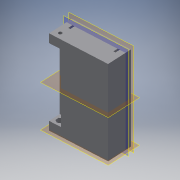
# Autodesk Inventor part: Caixa Painel
Saved by Autodesk Inventor 2019 (Build 230136000, 136)
## iProperties
Created: 2020-05-29
Part Number: Caixa Painel
Material: Generic
Document SubType Name: Modeling
Designer: luiza
Density: 1 g/cm^3
Appearance: Default
Categories: <MemberInstance><Categories><Category DisplayName="" Mnemonic="CABLEANDHARNESS" InternalName="e4a7e005-5e42-4d16-b293-125e7f0d0512"><Category DisplayName="" Mnemonic="CONNECTORS" InternalName="6f634eba-a678-4820-a31d-2c2d5ee6728e"><CategoryParameter DisplayName="" Mnemonic="REFDES" InternalName="c3740e8c-60ab-4d5d-8584-52b73222f2f0"/><Category DisplayName="" Mnemonic="DISCRETEWIRE" InternalName="9a3407de-09b2-4cdb-8c40-9708d5144a28"/></Category></Category></Categories><FamilyTemplate><FamilyTemplateParameters></FamilyTemplateParameters></FamilyTemplate><CategoryParameterMap><ParamToTemplateMap><ParamToTemplate CategoryParameter="//CategoryParameter[@InternalName='c3740e8c-60ab-4d5d-8584-52b73222f2f0']" ConstantValue=""/></ParamToTemplateMap></CategoryParameterMap></MemberInstance>
Author: luiza
Autodesk Inventor part; units mm, degrees
ref_plane "YZ Plane" through (0, 0, 0) normal (1, 0, 0) x (0, 1, 0)
ref_plane "XZ Plane" through (0, 0, 0) normal (0, 1, 0) x (-1, 0, 0)
ref_plane "XY Plane" through (0, 0, 0) normal (0, 0, 1) x (1, 0, 0)
ref_plane "Work Plane1" through (-1405.2046, 1188.2554, 32.7938) normal (0.0525168, 0, 0.99862) x (0, -1, 0)
sketch "Sketch1" plane through (-1405.2046, 1188.2554, 32.7938) normal (0.0525168, 0, 0.99862) x (0, -1, 0)
  line L0 (-58, 47) -> (58, 47)
  line L1 (72, 33) -> (72, -33)
  line L2 (58, -47) -> (-58, -47)
  line L3 (-72, -33) -> (-72, 33)
  line L4 (-65, 33) -> (-72, 33)
  line L5 (-58, 40) -> (-58, 47)
  arc A0 (-65, 33) -> (-58, 40) centre (-65, 40) ccw
  line L6 (0, 69.334) -> (0, -92.7299)
  line L7 (101.325, 0) -> (-113.3608, 0)
  line L8 (65, 33) -> (72, 33)
  line L9 (58, 40) -> (58, 47)
  arc A1 (58, 40) -> (65, 33) centre (65, 40) ccw
  line L10 (-65, -33) -> (-72, -33)
  line L11 (-58, -40) -> (-58, -47)
  arc A2 (-58, -40) -> (-65, -33) centre (-65, -40) ccw
  line L12 (58, -40) -> (58, -47)
  arc A3 (65, -33) -> (58, -40) centre (65, -40) ccw
  line L13 (65, -33) -> (72, -33)
  line L14 (75, -50) -> (75, 50)
  line L15 (75, 50) -> (-75, 50)
  line L16 (-75, 50) -> (-75, -50)
  line L17 (-75, -50) -> (75, -50)
  constraints: 36 end point, 15 symmetric about line, 8 point on circle, 4 centre point, 4 horizontal, 4 vertical, 1 coincident, 7 other
extrude "Extrusion1" add sketch "Sketch1" along normal blind 40 contours L5 A0 L4 L3 L7 L16 L15 L6 L0 | L6 L15 L14 L7 L1 L8 A1 L9 L0 | L6 L17 L16 L7 L3 L10 A2 L11 L2 | L2 L12 A3 L13 L1 L7 L14 L17 L6
sketch "Sketch2" plane through (-1403.1039, 1188.2554, 72.7386) normal (0.0525168, 0, 0.99862) x (0, -1, 0)
  line L0 (72, -33) -> (65, -33) projected
  arc A0 (65, -33) -> (58, -40) centre (65, -40) ccw projected
  line L1 (58, -40) -> (58, -47) projected
  line L2 (58, -47) -> (-58, -47) projected
  line L3 (-58, -47) -> (-58, -40) projected
  arc A1 (-58, -40) -> (-65, -33) centre (-65, -40) ccw projected
  line L4 (-65, -33) -> (-72, -33) projected
  line L5 (-72, -33) -> (-72, 33) projected
  line L6 (-72, 33) -> (-65, 33) projected
  arc A2 (-65, 33) -> (-58, 40) centre (-65, 40) ccw projected
  line L7 (-58, 40) -> (-58, 47) projected
  line L8 (-58, 47) -> (58, 47) projected
  line L9 (58, 47) -> (58, 40) projected
  arc A3 (58, 40) -> (65, 33) centre (65, 40) ccw projected
  line L10 (65, 33) -> (72, 33) projected
  line L11 (72, 33) -> (72, -33) projected
  line L12 (-75, 50) -> (75, 50)
  line L13 (75, 50) -> (75, -50)
  line L14 (75, -50) -> (-75, -50)
  line L15 (-75, -50) -> (-75, 50)
  point P0 (75, -40)
  constraints: 8 end point, 2 horizontal, 2 vertical, 4 other
extrude "Extrusion2" add sketch "Sketch2" along normal blind 3 contours L0 A0 L1 L2 L3 A1 L4 L5 L6 A2 L7 L8 L9 A3 L10 L11 | L12 L13 L14 L15
ref_plane "Work Plane2" through (-1404.6794, 1188.2554, 42.78) normal (-0.0525168, 0, -0.99862) x (0, -1, 0)
sketch "Sketch3" plane through (-1404.6794, 1188.2554, 42.78) normal (-0.0525168, 0, -0.99862) x (0, -1, 0)
  line L0 (72, -33) -> (72, 33) projected
  line L1 (-58, -47) -> (58, -47) projected
  line L2 (72, 0) -> (-85.4188, 0)
  line L3 (0, -47) -> (0, 56.7085)
  line L4 (-67.1246, 36.5) -> (-63.0716, 36.4992)
  line L5 (-69.1504, 40.0104) -> (-67.1246, 36.5) construction
  line L6 (-67.1232, 43.52) -> (-69.1504, 40.0104) construction
  line L7 (-63.0702, 43.5192) -> (-67.1232, 43.52)
  line L8 (-63.0716, 36.4992) -> (-61.0444, 40.0088)
  line L9 (-61.0444, 40.0088) -> (-63.0702, 43.5192)
  line L10 (-61.0444, 40.0088) -> (-77.9922, 40.0088)
  line L11 (-64.8068, 40.0088) -> (-83.3652, 40.0088) construction
  line L12 (-67.1232, 43.52) -> (-74.36, 43.52)
  line L13 (-67.1246, 36.5) -> (-75, 36.5)
  arc A0 (74.36, -43.52) -> (75, -40) centre (65, -40) ccw
  arc A1 (-75, -40) -> (-74.36, -43.52) centre (-65, -40) ccw
  arc A2 (-74.36, 43.52) -> (-75, 40) centre (-65, 40) ccw
  arc A3 (75, 40) -> (74.36, 43.52) centre (65, 40) ccw
  line L14 (63.0716, 36.4992) -> (61.0444, 40.0088)
  line L15 (61.0444, 40.0088) -> (63.0702, 43.5192)
  line L16 (69.1504, 40.0104) -> (67.1246, 36.5) construction
  line L17 (67.1232, 43.52) -> (69.1504, 40.0104) construction
  line L18 (67.1246, 36.5) -> (63.0716, 36.4992)
  line L19 (63.0702, 43.5192) -> (67.1232, 43.52)
  line L20 (61.0444, 40.0088) -> (77.9922, 40.0088)
  line L21 (67.1232, 43.52) -> (74.36, 43.52)
  line L22 (67.1246, 36.5) -> (75, 36.5)
  line L23 (-63.0716, -36.4992) -> (-61.0444, -40.0088)
  line L24 (-61.0444, -40.0088) -> (-63.0702, -43.5192)
  line L25 (-69.1504, -40.0104) -> (-67.1246, -36.5) construction
  line L26 (-67.1232, -43.52) -> (-69.1504, -40.0104) construction
  line L27 (-67.1246, -36.5) -> (-63.0716, -36.4992)
  line L28 (-63.0702, -43.5192) -> (-67.1232, -43.52)
  line L29 (-61.0444, -40.0088) -> (-77.9922, -40.0088)
  line L30 (-67.1232, -43.52) -> (-74.36, -43.52)
  line L31 (-67.1246, -36.5) -> (-75, -36.5)
  line L32 (63.0716, -36.4992) -> (61.0444, -40.0088)
  line L33 (61.0444, -40.0088) -> (63.0702, -43.5192)
  line L34 (69.1504, -40.0104) -> (67.1246, -36.5) construction
  line L35 (67.1246, -36.5) -> (63.0716, -36.4992)
  line L36 (63.0702, -43.5192) -> (67.1232, -43.52)
  line L37 (67.1232, -43.52) -> (69.1504, -40.0104) construction
  line L38 (67.1246, -36.5) -> (75, -36.5)
  line L39 (67.1232, -43.52) -> (74.36, -43.52)
  line L40 (61.0444, -40.0088) -> (77.9922, -40.0088)
  line L41 (-75, -40) -> (-75, -36.5)
  line L42 (-75, 36.5) -> (-75, 40)
  line L43 (75, 40) -> (75, 36.5)
  line L44 (75, -36.5) -> (75, -40)
  point P0 (1188.2554, -1404.9877)
  point P1 (64.8068, 40.0088)
  point P2 (-64.8068, -40.0088)
  point P3 (-65, -40)
  point P4 (65, -40)
  point P5 (64.8068, -40.0088)
  point P6 (65, -40)
  dimension "d27" = 7.02
  dimension "d28" = 7.02
  dimension "d29" = 7.02
  constraints: 86 end point, 34 symmetric about line, 8 point on circle, 7 centre point, 6 horizontal, 4 equal length, 2 midpoint, 2 parallel, 1 collinear, 1 vertical
  measures "d27" distance between parallel lines of L4 L7
  measures "d28" distance between parallel lines of L9 L5
  measures "d29" distance between parallel lines of L6 L8
extrude "Extrusion5" cut sketch "Sketch3" against normal blind 8
sketch "Sketch4" plane through (-1405.2046, 1188.2554, 32.7938) normal (-0.0525168, 0, -0.99862) x (0, -1, 0)
  line L0 (65, 33) -> (72, 33) projected
  line L1 (72, 33) -> (72, -33) projected
  line L2 (72, -33) -> (65, -33) projected
  arc A0 (65, -33) -> (58, -40) centre (65, -40) ccw projected
  line L3 (58, -40) -> (58, -47) projected
  line L4 (58, -47) -> (-58, -47) projected
  line L5 (-58, -47) -> (-58, -40) projected
  arc A1 (-58, -40) -> (-65, -33) centre (-65, -40) ccw projected
  line L6 (-65, -33) -> (-72, -33) projected
  line L7 (-72, -33) -> (-72, 33) projected
  line L8 (-72, 33) -> (-65, 33) projected
  arc A2 (-65, 33) -> (-58, 40) centre (-65, 40) ccw projected
  line L9 (-58, 40) -> (-58, 47) projected
  line L10 (-58, 47) -> (58, 47) projected
  line L11 (58, 47) -> (58, 40) projected
  arc A3 (58, 40) -> (65, 33) centre (65, 40) ccw projected
  circle A4 centre (-65, 40) radius 2
  circle A5 centre (65, 40) radius 2
  circle A6 centre (65, -40) radius 2
  circle A7 centre (-65, -40) radius 2
  point P0 (1188.2554, -1404.9877)
  dimension "d19" = 4
  dimension "d20" = 4
  dimension "d21" = 4
  dimension "d22" = 4
  constraints: 4 centre point
  measures "d19" diameter of A7
  measures "d20" diameter of A4
  measures "d21" diameter of A5
  measures "d22" diameter of A6
extrude "Extrusion6" cut sketch "Sketch4" against normal blind 24 contours A4 | A5 | A6 | A7
sketch "Sketch15" plane through (-1455.1356, 1113.2554, 35.4196) normal (0, -1, 0) x (0.99862, 0, -0.0525168)
  circle A0 centre (10, 33) radius 3
  line L0 (0, 40) -> (100, 40) projected
  line L1 (0, 0) -> (0, 40) projected
  point P0 (1454.9877, 41.0484)
  dimension "d74" = 7
  dimension "d75" = 6
  dimension "d76" = 10
  constraints: 1 centre point
  measures "d74" distance from line of L0 A0.centre
  measures "d75" diameter of A0
  measures "d76" distance from line of L1 A0.centre
extrude "Extrusion14" cut sketch "Sketch15" against normal through all
ref_plane "Work Plane7" through (-1438.1591, 1114.7554, 34.5268) normal (0, 1, 0) x (0.99862, 0, -0.0525168)
sketch "Sketch16" plane through (-1438.1591, 1114.7554, 34.5268) normal (0, 1, 0) x (0.99862, 0, -0.0525168)
  line L0 (-17, 0) -> (-17, -43) projected
  line L1 (-17, -43) -> (3, -43)
  line L2 (3, -43) -> (3, -23)
  line L3 (3, -23) -> (-17, -23)
  line L4 (-17, -23) -> (-17, -43)
  circle A0 centre (-7, -33) radius 3 projected
  dimension "d79" = 10
  dimension "d80" = 10
  constraints: 8 end point, 2 parallel, 1 horizontal, 1 perpendicular
  measures "d79" distance from line of L2 A0.centre
  measures "d80" distance from line of L3 A0.centre
extrude "Extrusion15" cut sketch "Sketch16" along normal up to surface (145.5 mm away)
sketch "Sketch17" plane through (-1438.1591, 1260.2554, 34.5268) normal (0, -1, 0) x (0.99862, 0, -0.0525168)
  line L0 (-17, 43) -> (3, 43) projected
  line L1 (-17, 23) -> (-17, 43) projected
  line L2 (-7, 23) -> (-14, 23) projected
  line L3 (3, 40) -> (3, 43) projected
  line L4 (3, 43) -> (3, 23)
  line L5 (-17, 23) -> (3, 23)
  line L6 (8, 18) -> (-17, 18)
  line L7 (8, 43) -> (8, 18)
  line L8 (83, 43) -> (-17, 43) projected
  line L9 (8, 43) -> (3, 43)
  line L10 (-17, 23) -> (-17, 18)
  line L11 (-17, 0) -> (-17, 43) projected
  dimension "d83" = 5
  constraints: 12 end point, 2 point on line, 1 collinear, 1 horizontal, 1 vertical
  measures "d83" distance between parallel lines of L4 L7
extrude "Extrusion16" add sketch "Sketch17" along normal up to surface (144 mm away) contours L8 L7 L6 L10 L5 L2 L4 L3
sketch "Sketch18" plane through (-1433.9553, 1260.2554, 57.3375) normal (0, -1, 0) x (0.99862, 0, -0.0525168)
  circle A0 centre (-10, 10) radius 3 projected
  circle A1 centre (-10, 10) radius 6.3509 construction
  line L0 (-10, 16.3509) -> (-4.5, 13.1754)
  line L1 (-4.5, 13.1754) -> (-4.5, 6.8246)
  line L2 (-4.5, 6.8246) -> (-10, 3.6491)
  line L3 (-10, 3.6491) -> (-15.5, 6.8246)
  line L4 (-15.5, 6.8246) -> (-15.5, 13.1754)
  line L5 (-15.5, 13.1754) -> (-10, 16.3509)
  line L6 (-15.5, 10) -> (-4.5, 10)
  line L7 (0, 0) -> (0, 20) projected
  line L8 (-20, 20) -> (0, 20) projected
  line L9 (-20, 0) -> (-20, 20) projected
  line L10 (-20, 0) -> (0, 0) projected
  circle A2 centre (-10, 10) radius 3 projected
  dimension "d89" = 11
  constraints: 14 end point, 6 point on circle, 3 equal length, 2 midpoint, 2 vertical, 1 centre point, 1 coincident, 1 parallel
  measures "d89" distance of L6.start L6.end
extrude "Extrusion17" add sketch "Sketch18" along normal blind 12
ref_plane "Work Plane8" through (-1455.1356, 1188.2554, 35.4196) normal (0, 1, 0) x (0.99862, 0, -0.0525168)
mirror "Mirror4" about plane through (-1455.1356, 1188.2554, 35.4196) normal (0, 1, 0) of "Extrusion17"
sketch "Sketch19" plane through (-1438.1591, 1114.7554, 34.5268) normal (0, 1, 0) x (0.99862, 0, -0.0525168)
  circle A0 centre (-7, -33) radius 3 projected
  line L0 (3, -43) -> (-17, -43) projected
  line L1 (3, -43) -> (3, -23) projected
  line L2 (3, -23) -> (-17, -23) projected
  line L3 (-17, -43) -> (-17, -23) projected
  point P0 (1437.9877, -41.0484)
extrude "Extrusion18" add sketch "Sketch19" along normal up to surface (1.5 mm away)
sketch "Sketch20" plane through (-1433.9553, 1128.2554, 57.3375) normal (0.0525168, 0, 0.99862) x (0.99862, 0, -0.0525168)
  arc A0 (-3.75, 66.129) -> (-13.25, 66.129) centre (-8.5, 66.129) ccw
  arc A1 (-13.25, 53.871) -> (-3.75, 53.871) centre (-8.5, 53.871) ccw
  line L0 (-3.75, 66.129) -> (-3.75, 53.871)
  line L1 (-13.25, 66.129) -> (-13.25, 53.871)
  line L2 (-20, 0) -> (0, 0) projected
  line L3 (0, 0) -> (0, 120) projected
  line L4 (0, 120) -> (-20, 120) projected
  line L5 (-20, 0) -> (-20, 120) projected
  line L6 (-17, 118) -> (-17, 2) projected
  line L7 (-17, 60) -> (0, 60)
  line L8 (-17, 118) -> (0, 118)
  line L9 (-8.5, 118) -> (-8.5, 0)
  line L10 (-3.75, 60) -> (-13.25, 60)
  line L11 (-8.5, 70.879) -> (-8.5, 49.121)
  arc A2 (-3.75, 93.387) -> (-13.25, 93.387) centre (-8.5, 93.387) ccw
  arc A3 (-13.25, 81.129) -> (-3.75, 81.129) centre (-8.5, 81.129) ccw
  line L12 (-3.75, 93.387) -> (-3.75, 81.129)
  line L13 (-13.25, 93.387) -> (-13.25, 81.129)
  line L14 (-3.75, 87.258) -> (-13.25, 87.258)
  line L15 (-8.5, 98.137) -> (-8.5, 76.379)
  arc A4 (-3.75, 38.871) -> (-13.25, 38.871) centre (-8.5, 38.871) ccw
  arc A5 (-13.25, 26.613) -> (-3.75, 26.613) centre (-8.5, 26.613) ccw
  line L16 (-3.75, 38.871) -> (-3.75, 26.613)
  line L17 (-13.25, 38.871) -> (-13.25, 26.613)
  line L18 (-3.75, 32.742) -> (-13.25, 32.742)
  line L19 (-8.5, 43.621) -> (-8.5, 21.863)
  point P0 (1434.9877, -1128.2554)
  point P1 (-20, 0)
  point P2 (-8.5, 60)
  point P3 (-8.5, 87.258)
  point P4 (-8.5, 32.742)
  dimension "d96" = 4.75
  dimension "d97" = 12.258
  dimension "d98" = 0
  dimension "d99" = 0
  dimension "d100" = 4.75
  dimension "d101" = 12.258
  dimension "d102" = 4.75
  dimension "d103" = 12.258
  dimension "d104" = 15
  dimension "d105" = 15
  constraints: 30 end point, 18 point on circle, 12 midpoint, 9 tangent, 7 vertical, 6 centre point, 3 parallel, 2 point on line, 1 horizontal, 1 other
  measures "d96" radius of A1
  measures "d97" distance of L1.start L1.end
  measures "d98" distance between parallel lines of L7 L10
  measures "d99" distance between parallel lines of L9 L11
  measures "d100" radius of A3
  measures "d101" distance of L13.start L13.end
  measures "d102" radius of A5
  measures "d103" distance of L17.start L17.end
  measures "d104" distance of A3.centre A0.centre
  measures "d105" distance of A4.centre A1.centre
extrude "Extrusion19" cut sketch "Sketch20" against normal up to next contours L0 L7 L9 A0 | L9 L7 L1 A0 | L0 A1 L9 L7 | A3 L13 L14 L9 | L9 L14 L12 A3 | L9 A1 L1 L7 | L14 L13 A2 L9 | L9 A2 L12 L14 | A4 L16 L18 L9 | L9 L18 L17 A4 | L18 L16 A5 L9 | L9 A5 L17 L18
body "Solid1"
